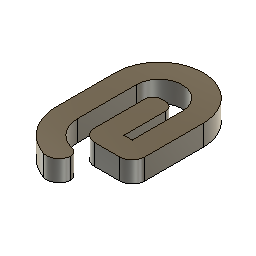
curtain-hook small v2 (Autodesk Fusion 360 design; units mm, degrees)
Autodesk Fusion 360 part; units mm, degrees
sketch "Skizze1" plane through (0, 0, 0) normal (0, 0, 1) x (1, 0, 0)
  line L0 (2.5, 0) -> (2.5, 5)
  line L1 (1.5, 6) -> (1, 6)
  line L2 (0, 5) -> (0, 0)
  line L3 (2.5, 0) -> (3.5, 0)
  line L4 (6, 0) -> (6, -1)
  line L5 (4.5, -2.5) -> (1.5, -2.5)
  line L6 (0, -1) -> (0, 0)
  line L7 (3.5, 0) -> (3.5, 5.9763)
  line L8 (6, 5.9763) -> (6, 0)
  line L9 (-4.5, 5.9763) -> (-4.5, -1)
  line L10 (-2, -1) -> (-2, 5.9763)
  arc A0 (2.5, 5) -> (1.5, 6) centre (1.5, 5) ccw
  arc A1 (1, 6) -> (0, 5) centre (1, 5) ccw
  arc A2 (0, -1) -> (1.5, -2.5) centre (1.5, -1) ccw
  arc A3 (4.5, -2.5) -> (6, -1) centre (4.5, -1) ccw
  arc A4 (-4.5, -1) -> (-0.5, -6.6569) centre (1.5, -1) ccw
  arc A5 (-2, -1) -> (0.663, -4.3985) centre (1.5, -1) ccw
  line L11 (1.5, -1) -> (1.5, -1.2605)
  line L12 (1.5, -5.4665) -> (1.5, -5.2426)
  arc A6 (1.5, -5.4665) -> (0.663, -4.3985) centre (0.4, -5.4665) ccw
  arc A7 (-0.5, -6.6569) -> (1.5, -5.2426) centre (0, -5.2426) ccw
  arc A8 (3.5, 5.9763) -> (-2, 5.9763) centre (0.75, 5.9763) ccw
  line L13 (1.7166, 5.9763) -> (0.7834, 5.9763)
  arc A9 (0, 0.7801) -> (2.5, 1.0265) centre (0.75, 5.9763) ccw
  arc A10 (6, 5.9763) -> (-4.5, 5.9763) centre (0.75, 5.9763) ccw
  line L14 (-2, 10.5) -> (-1.9142, 10.5)
  point P0 (0, 6)
  point P1 (0, -2.5)
  point P2 (-2, 8)
  point P3 (6, 10.5)
  point P4 (-4.5, 10.5)
  dimension "d1" = 2.5
  dimension "d2" = 6
  dimension "d3" = 2.5
  dimension "d4" = 6
  dimension "d5" = 2.5
  dimension "d10" = 2.5
  dimension "d11" = 1
  dimension "d13" = 1.5
  dimension "d14" = 1.5
  dimension "d17" = 1.1
  dimension "d18" = 1.5
  constraint vertical L0
  constraint horizontal L1
  constraint vertical L2
  constraint coincident L2.end L6.end
  constraint horizontal L3
  constraint vertical L4
  constraint horizontal L5
  constraint vertical L6
  constraint vertical L7
  constraint vertical L8
  constraint horizontal L14
  constraint vertical L9
  constraint vertical L10
  constraint tangent L1 A0
  constraint tangent L0 A0
  constraint coincident P2 L10
  constraint coincident P0 L2
  constraint coincident P0 L1
  constraint tangent L2 A1
  constraint tangent L1 A1
  constraint coincident P1 L6
  constraint coincident P1 L5
  constraint tangent L6 A2
  constraint tangent L5 A2
  constraint tangent L5 A3
  constraint tangent L4 A3
  constraint coincident P3 L14
  constraint coincident P4 L9
  constraint concentric A2 A5
  constraint tangent L10 A5
  constraint concentric A2 A4
  constraint tangent L9 A4
  constraint coincident A2.centre A4.centre
  constraint vertical L11
  constraint tangent A5 A6
  constraint tangent L12 A6
  constraint tangent L12 A7
  constraint tangent A4 A7
  constraint perpendicular L10 L13
  constraint concentric A8 A9
  constraint tangent L8 A9
  constraint coincident L2 A9.start
  constraint coincident L0 A9.end
  constraint concentric A9 A10
  constraint coincident A1 L13.end
  constraint coincident A0 L13.start
  constraint coincident A10 L14.end
  measures "d1" distance of L2.end L0.start
  measures "d2" distance of L2.end P0
  measures "d3" distance of L2.end P1
  measures "d4" distance of L2.end L4.start
  measures "d5" distance of L4.start L3.end
  measures "d10" distance of L14.start P4
  measures "d11" radius of A0
  measures "d13" radius of A2
  measures "d14" radius of A3
  measures "d17" radius of A6
  measures "d18" radius of A7
extrude "Extrusion1" add sketch "Skizze1" along normal blind 2.5 contours L0 L2 L3 L4 L5 L6 L7 L8 L9 L10 A2 A3 A4 A5 A6 A7 A8 A9 A10 | L0 L2 A0 A1 L13 A9 | L1 A0 A1 L13
sketch "Skizze2" plane through (0, 0, 2.5) normal (0, 0, 1) x (-1, 0, 0)
  line L0 (2, 1) -> (2, -5.9763)
  arc A0 (-3.5, -5.9763) -> (2, -5.9763) centre (-0.75, -5.9763) ccw
  line L1 (-3.5, -5.9763) -> (-3.5, 0)
  line L2 (-3.5, 0) -> (-2.5, 0)
  line L3 (-2.5, 0) -> (-2.5, -5)
  arc A1 (-2.5, -5) -> (-1.5, -6) centre (-1.5, -5) ccw
  line L4 (-1.5, -6) -> (-1, -6)
  arc A2 (-1, -6) -> (0, -5) centre (-1, -5) ccw
  line L5 (0, -5) -> (0, 1)
  arc A3 (0, 1) -> (-1.5, 2.5) centre (-1.5, 1) ccw
  line L6 (-1.5, 2.5) -> (-4.5, 2.5)
  arc A4 (-4.5, 2.5) -> (-6, 1) centre (-4.5, 1) ccw
  line L7 (-6, 1) -> (-6, -5.9763)
  arc A5 (-6, -5.9763) -> (4.5, -5.9763) centre (-0.75, -5.9763) ccw
  line L8 (4.5, -5.9763) -> (4.5, 1)
  arc A6 (4.5, 1) -> (0.5, 6.6569) centre (-1.5, 1) ccw
  arc A7 (0.5, 6.6569) -> (-1.4951, 5.3633) centre (0, 5.2426) ccw
  arc A8 (-1.4951, 5.3633) -> (-0.663, 4.3985) centre (-0.4, 5.4665) ccw
  arc A9 (2, 1) -> (-0.663, 4.3985) centre (-1.5, 1) ccw
